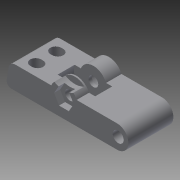
# Autodesk Inventor part: FelixOriginalBearingHolder
Saved by Autodesk Inventor 2015 SP1 (Build 190203100, 203)
## iProperties
Created: 2014-12-14
Part Number: FelixOriginalBearingHolder
Material: Generic
Document SubType Name: Modeling
Designer: Jack
Density: 1 g/cm^3
Appearance: Default
Author: Jack
Autodesk Inventor part; units mm, degrees
ref_plane "YZ Plane" through (0, 0, 0) normal (1, 0, 0) x (0, 1, 0)
ref_plane "XZ Plane" through (0, 0, 0) normal (0, 1, 0) x (-1, 0, 0)
sketch "Sketch1" plane through (0, 0, 0) normal (0, 0, 1) x (1, 0, 0)
  line L0 (0, 0) -> (1.4521, 9.38)
  line L1 (1.4521, 9.38) -> (50.35, 9.38)
  line L2 (50.35, 9.38) -> (50.35, 0)
  line L3 (50.35, 0) -> (0, 0)
  dimension "d7" = 81.2
  dimension "d8" = 50.35
  dimension "d9" = 9.38
  constraints: 8 end point, 2 perpendicular, 1 horizontal
  measures "d7" angle of L3 L0
  measures "d8" distance of L2.end L0.start
  measures "d9" distance of L1.end L2.end
extrude "Extrusion1" add sketch "Sketch1" along normal blind 18.5
fillet "Fillet1" radius 2.85 1 edges at (1.4521, 9.38, 9.25)
fillet "Fillet2" radius 1.85 1 edges at (0, 0, 9.25)
sketch "Sketch3" plane through (0, 0, 18.5) normal (0, 0, 1) x (1, 0, 0)
  line L0 (2.1584, 0) -> (50.35, 0) projected
  line L1 (50.35, 0) -> (50.35, 9.38) projected
  circle A0 centre (46.18, 4.8) radius 2.25
  point P0 (0, 0)
  dimension "d13" = 4.5
  dimension "d14" = 4.8
  dimension "d15" = 4.17
  constraints: 1 centre point
  measures "d13" diameter of A0
  measures "d14" distance from line of L0 A0.centre
  measures "d15" distance from line of L1 A0.centre
extrude "Extrusion2" cut sketch "Sketch3" against normal up to next
fillet "Fillet3" radius 4.6 2 edges at (50.35, 9.38, 9.25) (50.35, 0, 9.25)
sketch "Sketch5" plane through (0, 0, 18.5) normal (0, 0, 1) x (1, 0, 0)
  line L0 (45.75, 9.38) -> (3.8948, 9.38) projected
  arc A0 (29.0413, 9.38) -> (18.6587, 9.38) centre (23.85, 7.28) ccw
  point P0 (50.35, 4.6)
  point P1 (0, 0)
  dimension "d24" = 11.2
  dimension "d25" = 2.1
  dimension "d26" = 26.5
  constraints: 2 point on circle, 2 point on line, 1 centre point
  measures "d24" diameter of A0
  measures "d25" distance from line of L0 A0.centre
  measures "d26" horizontal distance of point (50.35, 4.6) A0.centre
extrude "Extrusion4" add sketch "Sketch5" against normal up to surface (18.5 mm away)
sketch "Sketch6" plane through (0, 0, 18.5) normal (0, 0, 1) x (1, 0, 0)
  arc A0 (29.0413, 9.38) -> (18.6587, 9.38) centre (23.85, 7.28) ccw projected
  line L0 (27.8915, 7.28) -> (25.8707, 3.78)
  line L1 (25.8707, 3.78) -> (21.8293, 3.78)
  line L2 (21.8293, 3.78) -> (19.8085, 7.28)
  line L3 (19.8085, 7.28) -> (21.8293, 10.78)
  line L4 (21.8293, 10.78) -> (25.8707, 10.78)
  line L5 (25.8707, 10.78) -> (27.8915, 7.28)
  point P0 (0, 0)
  dimension "d29" = 7
  constraints: 12 end point, 1 coincident, 1 horizontal, 13 other
  measures "d29" distance between parallel lines of L1 L4
extrude "Extrusion5" cut sketch "Sketch6" against normal blind 2.5
sketch "Sketch7" plane through (0, 0, 18.5) normal (0, 0, 1) x (1, 0, 0)
  arc A0 (29.0413, 9.38) -> (18.6587, 9.38) centre (23.85, 7.28) ccw projected
  circle A1 centre (23.85, 7.28) radius 2
  point P0 (0, 0)
  dimension "d32" = 4
  constraints: 1 centre point, 1 coincident
  measures "d32" diameter of A1
extrude "Extrusion6" cut sketch "Sketch7" against normal up to surface (18.5 mm away)
ref_plane "Work Plane1" through (0, 0, 13.37) normal (0, 0, 1) x (1, 0, 0)
sketch "Sketch8" plane through (0, 0, 13.37) normal (0, 0, 1) x (1, 0, 0)
  circle A0 centre (23.85, 7.28) radius 2 projected
  circle A1 centre (23.85, 7.28) radius 8
  point P0 (0, 0)
  dimension "d36" = 16
  constraints: 1 centre point, 1 coincident
  measures "d36" diameter of A1
extrude "Extrusion7" cut sketch "Sketch8" against normal blind 7
sketch "Sketch9" plane through (0, 0, 18.5) normal (0, 0, 1) x (1, 0, 0)
  line L0 (45.75, 9.38) -> (29.0413, 9.38) projected
  arc A0 (29.0413, 9.38) -> (18.6587, 9.38) centre (23.85, 7.28) ccw projected
  circle A1 centre (23.85, 17.79) radius 7.6
  point P0 (0, 0)
  dimension "d39" = 15.2
  dimension "d40" = 8.41
  constraints: 1 centre point, 1 vertical alignment
  measures "d39" diameter of A1
  measures "d40" distance from line of L0 A1.centre
extrude "Extrusion8" cut sketch "Sketch9" against normal blind 4.5
sketch "Sketch10" plane through (0, 0, 0) normal (0, 0, -1) x (-1, 0, 0)
  circle A0 centre (-23.85, 7.28) radius 2 projected
  arc A1 (-18.6587, 9.38) -> (-29.0413, 9.38) centre (-23.85, 7.28) ccw projected
  circle A2 centre (-23.85, 7.28) radius 3.6
  point P0 (0, 0)
  dimension "d43" = 7.2
  constraints: 1 centre point, 1 coincident
  measures "d43" diameter of A2
extrude "Extrusion9" cut sketch "Sketch10" against normal blind 5
sketch "Sketch11" plane through (3.8948, 9.38, 18.5) normal (0, 1, 0) x (1, 0, 0)
  line L0 (0, 18.5) -> (14.7638, 18.5) projected
  line L1 (14.7638, 0) -> (0, 0) projected
  line L2 (3.4252, 13.2) -> (4.2552, 13.2) construction
  line L3 (3.4252, 10.95) -> (4.2552, 10.95)
  line L4 (4.2552, 15.45) -> (3.4252, 15.45)
  arc A0 (3.4252, 15.45) -> (3.4252, 10.95) centre (3.4252, 13.2) ccw
  arc A1 (4.2552, 10.95) -> (4.2552, 15.45) centre (4.2552, 13.2) ccw
  line L5 (3.4252, 4.9) -> (4.2552, 4.9) construction
  line L6 (3.4252, 2.65) -> (4.2552, 2.65)
  line L7 (4.2552, 7.15) -> (3.4252, 7.15)
  arc A2 (3.4252, 7.15) -> (3.4252, 2.65) centre (3.4252, 4.9) ccw
  arc A3 (4.2552, 2.65) -> (4.2552, 7.15) centre (4.2552, 4.9) ccw
  line L8 (46.4552, 0) -> (46.4552, 18.5) projected
  point P0 (-3.8948, 18.5)
  point P1 (3.8402, 13.2)
  point P2 (3.8402, 4.9)
  dimension "d46" = 4.5
  dimension "d47" = 0.83
  dimension "d48" = 4.9
  dimension "d49" = 5.3
  dimension "d50" = 42.2
  constraints: 16 end point, 8 point on circle, 8 tangent, 4 centre point, 4 parallel, 2 midpoint, 1 equal radius, 1 horizontal, 1 vertical alignment
  measures "d46" diameter of A1
  measures "d47" distance of L2.start L2.end
  measures "d48" distance from line of L1 point (3.84, 4.9)
  measures "d49" distance from line of L0 point (3.84, 13.2)
  measures "d50" distance from line of L8 L5.end
extrude "Extrusion10" cut sketch "Sketch11" against normal up to next
sketch "Sketch12" plane through (2.1584, 0, 0) normal (0, -1, 0) x (1, 0, 0)
  arc A0 (5.9916, 3.05) -> (5.9916, 7.55) centre (5.9916, 5.3) ccw projected
  line L0 (5.9916, 3.05) -> (5.1616, 3.05) projected
  arc A1 (5.1616, 7.55) -> (5.1616, 3.05) centre (5.1616, 5.3) ccw projected
  line L1 (5.1616, 7.55) -> (5.9916, 7.55) projected
  arc A2 (5.9916, 11.35) -> (5.9916, 15.85) centre (5.9916, 13.6) ccw projected
  line L2 (5.9916, 11.35) -> (5.1616, 11.35) projected
  arc A3 (5.1616, 15.85) -> (5.1616, 11.35) centre (5.1616, 13.6) ccw projected
  line L3 (5.1616, 15.85) -> (5.9916, 15.85) projected
  line L4 (10.033, 13.6) -> (8.0123, 10.1)
  line L5 (8.0123, 10.1) -> (3.9708, 10.1)
  line L6 (3.9708, 10.1) -> (1.9501, 13.6)
  line L7 (1.9501, 13.6) -> (3.9708, 17.1)
  line L8 (3.9708, 17.1) -> (8.0123, 17.1)
  line L9 (8.0123, 17.1) -> (10.033, 13.6)
  line L10 (1.1201, 13.6) -> (3.1408, 17.1)
  line L11 (3.1408, 17.1) -> (7.1823, 17.1)
  line L12 (7.1823, 17.1) -> (9.203, 13.6)
  line L13 (9.203, 13.6) -> (7.1823, 10.1)
  line L14 (7.1823, 10.1) -> (3.1408, 10.1)
  line L15 (3.1408, 10.1) -> (1.1201, 13.6)
  line L16 (10.033, 5.3) -> (8.0123, 1.8)
  line L17 (8.0123, 1.8) -> (3.9708, 1.8)
  line L18 (3.9708, 1.8) -> (1.9501, 5.3)
  line L19 (1.9501, 5.3) -> (3.9708, 8.8)
  line L20 (3.9708, 8.8) -> (8.0123, 8.8)
  line L21 (8.0123, 8.8) -> (10.033, 5.3)
  line L22 (1.1201, 5.3) -> (3.1408, 8.8)
  line L23 (3.1408, 8.8) -> (7.1823, 8.8)
  line L24 (7.1823, 8.8) -> (9.203, 5.3)
  line L25 (9.203, 5.3) -> (7.1823, 1.8)
  line L26 (7.1823, 1.8) -> (3.1408, 1.8)
  line L27 (3.1408, 1.8) -> (1.1201, 5.3)
  point P0 (-2.1584, 0)
  dimension "d53" = 7
  constraints: 48 end point, 4 coincident, 4 horizontal, 3 equal length, 52 other
  measures "d53" distance between parallel lines of L14 L11
extrude "Extrusion11" cut sketch "Sketch12" against normal blind 3.9 contours L0 A1 L1 A0 | L2 A3 L3 A2 | L4 L5 L13 L12 L8 L9 | L5 L6 L7 L8 L12 L13 | L14 L15 L10 L11 L7 L6 | L16 L17 L25 L24 L20 L21 | L17 L18 L19 L20 L24 L25 | L26 L27 L22 L23 L19 L18
body "Solid1"
